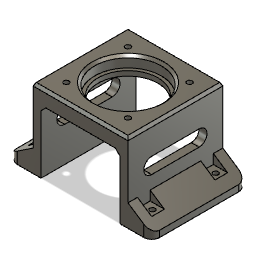
bearing_support (Autodesk Fusion 360 design; units mm, degrees)
Autodesk Fusion 360 part; units mm, degrees
sketch "Sketch1" plane through (0, 0, 0) normal (0, 0, 1) x (1, 0, 0)
  line L0 (-45, -42) -> (-45, -38)
  line L1 (-45, -38) -> (-30, -38)
  line L2 (-30, -38) -> (-30, 8)
  line L3 (-30, 8) -> (30, 8)
  line L4 (30, 8) -> (30, -38)
  line L5 (30, -38) -> (45, -38)
  line L6 (45, -38) -> (45, -42)
  line L7 (45, -42) -> (25, -42)
  line L8 (25, -42) -> (25, -2)
  line L9 (25, -2) -> (-25, -2)
  line L10 (-25, -2) -> (-25, -42)
  line L11 (-25, -42) -> (-45, -42)
  dimension "d1" = 60
  dimension "d2" = 30
  dimension "d3" = 4
  dimension "d4" = 4
  dimension "d5" = 5
  dimension "d6" = 5
  dimension "d7" = 10
  dimension "d8" = 15
  dimension "d9" = 15
  dimension "d24" = 46
  dimension "d25" = 46
  constraint vertical L0
  constraint perpendicular L0 L1
  constraint perpendicular L1 L2
  constraint perpendicular L2 L3
  constraint perpendicular L3 L4
  constraint perpendicular L4 L5
  constraint perpendicular L5 L6
  constraint perpendicular L6 L7
  constraint perpendicular L7 L8
  constraint perpendicular L8 L9
  constraint perpendicular L9 L10
  constraint perpendicular L0 L11
  measures "d1" distance of L2.end L3.end
  measures "d2" distance of origin L4
  measures "d3" distance of L5.end L6.end
  measures "d4" distance of L0.start L0.end
  measures "d5" distance of L4 L8
  measures "d6" distance of L2 L10
  measures "d7" distance of L3 L9
  measures "d8" distance of L4.end L5.end
  measures "d9" distance of L0.end L1.end
  measures "d24" distance of L3.end L4.end
  measures "d25" distance of L1.end L2.end
extrude "Extrude1" add sketch "Sketch1" along normal blind 60
sketch "Sketch2" plane through (0, 8, 0) normal (0, 1, 0) x (-1, 0, 0)
  line L0 (-30, 0) -> (30, 0)
  line L1 (30, 0) -> (30, 60)
  line L2 (30, 60) -> (-30, 60)
  line L3 (-30, 60) -> (-30, 0)
  circle A0 centre (0, 30) radius 21.1
  dimension "d14" = 42.2
  dimension "d15" = 30
  dimension "d16" = 30
  measures "d14" diameter of A0
  measures "d15" distance of L0 A0.centre
  measures "d16" distance of L3 A0.centre
extrude "Extrude2" cut sketch "Sketch2" against normal blind 7 contours A0
sketch "Sketch3" plane through (0, 1, 0) normal (0, 1, 0) x (-1, 0, 0)
  circle A0 centre (0, 30) radius 21.1
  circle A1 centre (0, 30) radius 19
  dimension "d20" = 38
  constraint concentric A0 A1
  measures "d20" diameter of A1
extrude "Extrude3" cut sketch "Sketch3" against normal up to surface (3 mm away) contours A1
chamfer "Chamfer1" distance 10 distance2 15 1 edges at (-30, -38, 30) measured on face at (-30, -22.6667, 40)
chamfer "Chamfer2" distance 15 distance2 10 1 edges at (30, -38, 30) measured on face at (35, -38, 20)
chamfer "Chamfer3" distance 1.5 angle 45 1 edges at (19.6721, 8, 37.6301)
chamfer "Chamfer4" distance 2 distance2 1 2 edges at (0, 8, 0) (0, 8, 60) measured on face at (33.3323, -36.0007, 0) measured on face at (33.3323, -36.0007, 60)
chamfer "Chamfer5" distance 2 distance2 1 1 edges at (30, 8, 30) measured on face at (30, -5.334, 40)
chamfer "Chamfer6" distance 1 distance2 2 1 edges at (-30, 8, 30) measured on face at (-27.5333, 8, 30)
chamfer "Chamfer7" distance 3 angle 45 2 edges at (25, -2, 30) (-25, -2, 30)
sketch "Sketch4" plane through (0, 8, 0) normal (0, 1, 0) x (-1, 0, 0)
  circle A0 centre (0, 30) radius 22.6
  line L0 (29, 1) -> (29, 59)
  line L1 (29, 59) -> (-29, 59)
  line L2 (-29, 59) -> (-29, 1)
  line L3 (-29, 1) -> (29, 1)
  circle A1 centre (-19.5, 10.5) radius 1.65
  circle A2 centre (19.5, 10.5) radius 1.65
  circle A3 centre (19.5, 49.5) radius 1.65
  circle A4 centre (-19.5, 49.5) radius 1.65
  dimension "d40" = 3.3
  dimension "d41" = 19.5
  dimension "d42" = 19.5
  dimension "d44" = 360
  measures "d40" diameter of A1
  measures "d41" vertical distance of A0.centre A1.centre
  measures "d42" horizontal distance of A0.centre A1.centre
extrude "Extrude4" cut sketch "Sketch4" against normal blind 15 contours A1 | A2 | A3 | A4
sketch "Sketch5" plane through (0, -2, 0) normal (0, -1, 0) x (1, 0, 0)
  circle A0 centre (-19.5, 10.5) radius 1.65
  circle A1 centre (-19.5, 49.5) radius 1.65
  circle A2 centre (19.5, 10.5) radius 1.65
  circle A3 centre (19.5, 49.5) radius 1.65
  circle A4 centre (0, 30) radius 19
  line L0 (-22, 60) -> (-22, 0)
  line L1 (-22, 0) -> (22, 0)
  line L2 (22, 0) -> (22, 60)
  line L3 (22, 60) -> (-22, 60)
  circle A5 centre (19.5, 49.5) radius 4
  circle A6 centre (-19.5, 49.5) radius 4
  circle A7 centre (-19.5, 10.5) radius 4
  circle A8 centre (19.5, 10.5) radius 4
  dimension "d47" = 8
  dimension "d49" = 360
  constraint concentric A3 A5
  measures "d47" diameter of A5
extrude "Extrude5" cut sketch "Sketch5" along normal blind -2 and the other way blind -2 contours L0 A6 | L0 A6 | L2 A5 | L2 A5 | L0 A7 | L0 A7 | L2 A8 | L2 A8
sketch "Sketch6" plane through (0, -42, 0) normal (0, -1, 0) x (1, 0, 0)
  line L0 (25, 0) -> (45, 0)
  line L1 (45, 0) -> (45, 60)
  line L2 (45, 60) -> (25, 60)
  line L3 (25, 60) -> (25, 0)
  circle A0 centre (35.5, 50) radius 1.65
  circle A1 centre (35.5, 10) radius 1.65
  circle A2 centre (-35.5, 10) radius 1.65
  circle A3 centre (-35.5, 50) radius 1.65
  arc A4 (-22, 46.3775) -> (-22, 52.6225) centre (-19.5, 49.5) ccw
  arc A5 (22, 52.6225) -> (22, 46.3775) centre (19.5, 49.5) ccw
  arc A6 (22, 13.6225) -> (22, 7.3775) centre (19.5, 10.5) ccw
  arc A7 (-22, 7.3775) -> (-22, 13.6225) centre (-19.5, 10.5) ccw
  dimension "d54" = 3.3
  dimension "d55" = 10
  dimension "d57" = 3.3
  dimension "d59" = 10
  dimension "d60" = 3.3
  dimension "d61" = 10
  dimension "d63" = 3.3
  dimension "d64" = 10
  dimension "d66" = 16
  dimension "d67" = 16
  dimension "d68" = 16
  dimension "d69" = 16
  measures "d54" diameter of A0
  measures "d55" distance of L2 A0.centre
  measures "d57" diameter of A1
  measures "d59" distance of L0 A1.centre
  measures "d60" diameter of A2
  measures "d61" distance of L0 A2.centre
  measures "d63" diameter of A3
  measures "d64" distance of L2 A3.centre
  measures "d66" horizontal distance of A3.centre A4.centre
  measures "d67" horizontal distance of A0.centre A5.centre
  measures "d68" horizontal distance of A1.centre A6.centre
  measures "d69" horizontal distance of A2.centre A7.centre
extrude "Extrude6" cut sketch "Sketch6" against normal blind 25 contours A0 | A1 | A2 | A3
sketch "Sketch7" plane through (45, 0, 0) normal (1, 0, 0) x (0, 0, -1)
  line L0 (0, -42) -> (0, -38)
  line L1 (0, -38) -> (-60, -38)
  line L2 (-60, -38) -> (-60, -42)
  line L3 (-60, -42) -> (0, -42)
  line L4 (-54, -28) -> (-46, -28)
  line L5 (-46, -28) -> (-46, -34)
  line L6 (-46, -34) -> (-54, -34)
  line L7 (-54, -34) -> (-54, -28)
  line L8 (-14, -28) -> (-6, -28)
  line L9 (-6, -28) -> (-6, -34)
  line L10 (-6, -34) -> (-14, -34)
  line L11 (-14, -34) -> (-14, -28)
  dimension "d72" = 8
  dimension "d73" = 6
  dimension "d74" = 8
  dimension "d75" = 8
  dimension "d76" = 8
  dimension "d77" = 6
  constraint horizontal L4
  constraint vertical L5
  constraint horizontal L6
  constraint vertical L7
  constraint horizontal L8
  constraint vertical L9
  constraint horizontal L10
  constraint vertical L11
  measures "d72" distance of L3 L6
  measures "d73" distance of L4.start L6.end
  measures "d74" distance of L4.start L4.end
  measures "d75" distance of L3 L10
  measures "d76" distance of L8.start L8.end
  measures "d77" distance of L8.end L9.end
extrude "Extrude7" cut sketch "Sketch7" against normal blind 15 contours L4 L5 L6 L7 | L8 L9 L10 L11
sketch "Sketch8" plane through (-45, 0, 0) normal (-1, 0, 0) x (0, 0, 1)
  line L0 (0, -38) -> (0, -42)
  line L1 (0, -42) -> (60, -42)
  line L2 (60, -42) -> (60, -38)
  line L3 (60, -38) -> (0, -38)
  line L4 (6, -28) -> (14, -28)
  line L5 (14, -28) -> (14, -34)
  line L6 (14, -34) -> (6, -34)
  line L7 (6, -34) -> (6, -28)
  line L8 (46, -28) -> (54, -28)
  line L9 (54, -28) -> (54, -34)
  line L10 (54, -34) -> (46, -34)
  line L11 (46, -34) -> (46, -28)
  dimension "d80" = 8
  dimension "d81" = 8
  dimension "d82" = 6
  dimension "d83" = 8
  dimension "d84" = 8
  dimension "d85" = 6
  constraint horizontal L4
  constraint vertical L5
  constraint horizontal L6
  constraint vertical L7
  constraint horizontal L8
  constraint vertical L9
  constraint horizontal L10
  constraint vertical L11
  measures "d80" distance of L1 L6
  measures "d81" distance of L4.start L4.end
  measures "d82" distance of L4.start L6.end
  measures "d83" distance of L1 L10
  measures "d84" distance of L8.start L8.end
  measures "d85" distance of L8.end L9.end
extrude "Extrude8" cut sketch "Sketch8" against normal blind 15 contours L4 L5 L6 L7 | L8 L9 L10 L11
fillet "Fillet1" radius 5 4 edges at (-45, -40, 0) (45, -40, 0) (45, -40, 60) (-45, -40, 60)
sketch "Sketch9" plane through (30, 0, 0) normal (1, 0, 0) x (0, 0, -1)
  line L0 (0, 6) -> (-60, 6)
  line L1 (-60, 6) -> (-60, -28)
  line L2 (-60, -28) -> (-54, -28)
  line L3 (-54, -28) -> (-54, -34)
  line L4 (-54, -34) -> (-46, -34)
  line L5 (-46, -34) -> (-46, -28)
  line L6 (-46, -28) -> (-14, -28)
  line L7 (-14, -28) -> (-14, -34)
  line L8 (-14, -34) -> (-6, -34)
  line L9 (-6, -34) -> (-6, -28)
  line L10 (-6, -28) -> (0, -28)
  line L11 (0, -28) -> (0, 6)
  line L12 (-45, -20) -> (-15, -20)
  arc A0 (-15, -20) -> (-15, -10) centre (-15, -15) ccw
  line L13 (-15, -10) -> (-45, -10)
  arc A1 (-45, -10) -> (-45, -20) centre (-45, -15) ccw
  line L14 (-45, -15) -> (-15, -15) construction
  dimension "d89" = 30
  dimension "d90" = 15
  dimension "d91" = 15
  constraint tangent L12 A0
  constraint tangent A0 L13
  constraint parallel L12 L13
  constraint tangent L13 A1
  constraint tangent L12 A1
  constraint horizontal L14
  measures "d89" distance of A1.centre A0.centre
  measures "d90" distance of L11 A0.centre
  measures "d91" distance of origin L14
extrude "Extrude9" cut sketch "Sketch9" against normal up to surface (60 mm away) contours L12 A0 L13 A1
equation "d1 = main"
equation "d2 = d1 / 2"
equation "d3 = leg_thickness"
equation "d4 = leg_thickness"
equation "d6 = d5"
equation "d8 = leg"
equation "d9 = leg"
equation "main = 60 mm"
equation "d11 = main"
equation "bearing_od = 42.2 mm"
equation "d14 = bearing_od"
equation "d15 = main / 2"
equation "d16 = main / 2"
equation "bearing_thickness = 7 mm"
equation "d18 = -bearing_thickness"
equation "height = 46 mm"
equation "d24 = height"
equation "d25 = height"
equation "leg = 15 mm"
equation "d28 = leg"
equation "d29 = leg"
equation "leg_thickness = 4 mm"
equation "d41 = d42"
equation "d57 = d54"
equation "d59 = d55"
equation "d60 = d54"
equation "d61 = d55"
equation "d63 = d54"
equation "d64 = d55"
equation "d66 = d67"
equation "d68 = d67"
equation "d69 = d67"
equation "d75 = d72"
equation "d76 = d74"
equation "d77 = d73"
